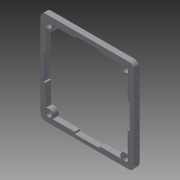
# Autodesk Inventor part: keyboard_space_cad
Saved by Autodesk Inventor 2014 (Build 180170000, 170)
## iProperties
Created: 2014-07-19
Part Number: keyboard_space_cad
Material: Generic
Document SubType Name: Modeling
Designer: james
Density: 1 g/cm^3
Appearance: Default
Author: james
Autodesk Inventor part; units mm, degrees
ref_plane "YZ Plane" through (0, 0, 0) normal (1, 0, 0) x (0, 1, 0)
ref_plane "XZ Plane" through (0, 0, 0) normal (0, 1, 0) x (-1, 0, 0)
ref_plane "XY Plane" through (0, 0, 0) normal (0, 0, 1) x (1, 0, 0)
sketch "Baseline" plane through (0, 0, 0) normal (0, 1, 0) x (-1, 0, 0)
  line L0 (61.0726, -11.6756) -> (16.1384, -11.6756)
  spline S0 degree 3 poles (16.1384, -11.6756) (13.8101, -11.6756) (11.9051, -13.5806) (11.9051, -15.909) knots 1 1 1 1 2 2 2 2
  line L1 (16.1384, -11.6756) -> (13.8101, -11.6756) construction
  line L2 (13.8101, -11.6756) -> (11.9051, -13.5806) construction
  line L3 (11.9051, -13.5806) -> (11.9051, -15.909) construction
  line L4 (11.9051, -15.909) -> (11.9051, -60.661)
  spline S1 degree 3 poles (11.9051, -60.661) (11.9051, -62.9893) (13.8101, -64.8943) (16.1384, -64.8943) knots 3 3 3 3 4 4 4 4
  line L5 (11.9051, -60.661) -> (11.9051, -62.9893) construction
  line L6 (11.9051, -62.9893) -> (13.8101, -64.8943) construction
  line L7 (13.8101, -64.8943) -> (16.1384, -64.8943) construction
  line L8 (16.1384, -64.8943) -> (61.0726, -64.8943)
  spline S2 degree 3 poles (61.0726, -64.8943) (63.4009, -64.8943) (65.3059, -62.9893) (65.3059, -60.661) knots 5 5 5 5 6 6 6 6
  line L9 (61.0726, -64.8943) -> (63.4009, -64.8943) construction
  line L10 (63.4009, -64.8943) -> (65.3059, -62.9893) construction
  line L11 (65.3059, -62.9893) -> (65.3059, -60.661) construction
  line L12 (65.3059, -60.661) -> (65.3059, -15.909)
  spline S3 degree 3 poles (65.3059, -15.909) (65.3059, -13.5806) (63.4009, -11.6756) (61.0726, -11.6756) knots 7 7 7 7 8 8 8 8
  line L13 (65.3059, -15.909) -> (65.3059, -13.5806) construction
  line L14 (65.3059, -13.5806) -> (63.4009, -11.6756) construction
  line L15 (63.4009, -11.6756) -> (61.0726, -11.6756) construction
  spline S4 degree 3 poles (59.9166, -15.3859) (59.9168, -15.3857) (59.9171, -15.3855) (59.9173, -15.3853) knots 0 0 0 0 1 1 1 1
  line L16 (59.9166, -15.3859) -> (59.9168, -15.3857) construction
  line L17 (59.9168, -15.3857) -> (59.9171, -15.3855) construction
  line L18 (59.9171, -15.3855) -> (59.9173, -15.3853) construction
  line L19 (59.9173, -15.3853) -> (59.9173, -15.3854)
  spline S5 degree 3 poles (59.9173, -15.3854) (60.1545, -15.1997) (60.4494, -15.0845) (60.7739, -15.0845) (61.5454, -15.0845) (62.1709, -15.7099) (62.1709, -16.4815) (62.1709, -16.7261) (62.1024, -16.9527) (61.9919, -17.1527) knots 2 2 2 2 3 3 3 4 4 4 5 5 5 5
  line L20 (59.9173, -15.3854) -> (60.1545, -15.1997) construction
  line L21 (60.1545, -15.1997) -> (60.4494, -15.0845) construction
  line L22 (60.4494, -15.0845) -> (60.7739, -15.0845) construction
  line L23 (60.7739, -15.0845) -> (61.5454, -15.0845) construction
  line L24 (61.5454, -15.0845) -> (62.1709, -15.7099) construction
  line L25 (62.1709, -15.7099) -> (62.1709, -16.4815) construction
  line L26 (62.1709, -16.4815) -> (62.1709, -16.7261) construction
  line L27 (62.1709, -16.7261) -> (62.1024, -16.9527) construction
  line L28 (62.1024, -16.9527) -> (61.9919, -17.1527) construction
  line L29 (61.9919, -17.1527) -> (61.9919, -17.1527)
  spline S6 degree 3 poles (61.9919, -17.1527) (61.9084, -17.3039) (61.7991, -17.4365) (61.6678, -17.5468) knots 7 7 7 7 8 8 8 8
  line L30 (61.9919, -17.1527) -> (61.9084, -17.3039) construction
  line L31 (61.9084, -17.3039) -> (61.7991, -17.4365) construction
  line L32 (61.7991, -17.4365) -> (61.6678, -17.5468) construction
  spline S7 degree 3 poles (61.6678, -17.5468) (61.6518, -17.5604) (61.6359, -17.5739) (61.6194, -17.5867) knots 8 8 8 8 9 9 9 9
  line L33 (61.6678, -17.5468) -> (61.6518, -17.5604) construction
  line L34 (61.6518, -17.5604) -> (61.6359, -17.5739) construction
  line L35 (61.6359, -17.5739) -> (61.6194, -17.5867) construction
  spline S8 degree 3 poles (61.6194, -17.5867) (61.583, -17.6147) (61.5464, -17.6415) (61.5073, -17.6658) knots 9 9 9 9 10 10 10 10
  line L36 (61.6194, -17.5867) -> (61.583, -17.6147) construction
  line L37 (61.583, -17.6147) -> (61.5464, -17.6415) construction
  line L38 (61.5464, -17.6415) -> (61.5073, -17.6658) construction
  spline S9 degree 3 poles (61.5073, -17.6658) (61.4604, -17.6954) (61.4112, -17.7214) (61.3608, -17.7453) knots 10 10 10 10 11 11 11 11
  line L39 (61.5073, -17.6658) -> (61.4604, -17.6954) construction
  line L40 (61.4604, -17.6954) -> (61.4112, -17.7214) construction
  line L41 (61.4112, -17.7214) -> (61.3608, -17.7453) construction
  spline S10 degree 3 poles (61.3608, -17.7453) (61.3302, -17.7595) (61.2994, -17.7722) (61.2677, -17.7842) knots 11 11 11 11 12 12 12 12
  line L42 (61.3608, -17.7453) -> (61.3302, -17.7595) construction
  line L43 (61.3302, -17.7595) -> (61.2994, -17.7722) construction
  line L44 (61.2994, -17.7722) -> (61.2677, -17.7842) construction
  spline S11 degree 3 poles (61.2677, -17.7842) (61.2113, -17.8059) (61.1534, -17.824) (61.0936, -17.8382) knots 12 12 12 12 13 13 13 13
  line L45 (61.2677, -17.7842) -> (61.2113, -17.8059) construction
  line L46 (61.2113, -17.8059) -> (61.1534, -17.824) construction
  line L47 (61.1534, -17.824) -> (61.0936, -17.8382) construction
  spline S12 degree 3 poles (61.0936, -17.8382) (61.0698, -17.8439) (61.0461, -17.8491) (61.0217, -17.8535) knots 13 13 13 13 14 14 14 14
  line L48 (61.0936, -17.8382) -> (61.0698, -17.8439) construction
  line L49 (61.0698, -17.8439) -> (61.0461, -17.8491) construction
  line L50 (61.0461, -17.8491) -> (61.0217, -17.8535) construction
  spline S13 degree 3 poles (61.0217, -17.8535) (60.9411, -17.8682) (60.8589, -17.8785) (60.7739, -17.8785) (60.0023, -17.8785) (59.3769, -17.253) (59.3769, -16.4815) (59.3769, -16.3956) (59.387, -16.3124) (59.4021, -16.2311) knots 14 14 14 14 15 15 15 16 16 16 17 17 17 17
  line L51 (61.0217, -17.8535) -> (60.9411, -17.8682) construction
  line L52 (60.9411, -17.8682) -> (60.8589, -17.8785) construction
  line L53 (60.8589, -17.8785) -> (60.7739, -17.8785) construction
  line L54 (60.7739, -17.8785) -> (60.0023, -17.8785) construction
  line L55 (60.0023, -17.8785) -> (59.3769, -17.253) construction
  line L56 (59.3769, -17.253) -> (59.3769, -16.4815) construction
  line L57 (59.3769, -16.4815) -> (59.3769, -16.3956) construction
  line L58 (59.3769, -16.3956) -> (59.387, -16.3124) construction
  line L59 (59.387, -16.3124) -> (59.4021, -16.2311) construction
  spline S14 degree 3 poles (59.4021, -16.2311) (59.4052, -16.2142) (59.4075, -16.1974) (59.4112, -16.1808) knots 17 17 17 17 18 18 18 18
  line L60 (59.4021, -16.2311) -> (59.4052, -16.2142) construction
  line L61 (59.4052, -16.2142) -> (59.4075, -16.1974) construction
  line L62 (59.4075, -16.1974) -> (59.4112, -16.1808) construction
  spline S15 degree 3 poles (59.4112, -16.1808) (59.4271, -16.11) (59.4487, -16.0414) (59.475, -15.9752) knots 18 18 18 18 19 19 19 19
  line L63 (59.4112, -16.1808) -> (59.4271, -16.11) construction
  line L64 (59.4271, -16.11) -> (59.4487, -16.0414) construction
  line L65 (59.4487, -16.0414) -> (59.475, -15.9752) construction
  spline S16 degree 3 poles (59.475, -15.9752) (59.486, -15.9472) (59.4982, -15.9203) (59.5108, -15.8933) knots 19 19 19 19 20 20 20 20
  line L66 (59.475, -15.9752) -> (59.486, -15.9472) construction
  line L67 (59.486, -15.9472) -> (59.4982, -15.9203) construction
  line L68 (59.4982, -15.9203) -> (59.5108, -15.8933) construction
  spline S17 degree 3 poles (59.5108, -15.8933) (59.5311, -15.8506) (59.5537, -15.8095) (59.5781, -15.7694) knots 20 20 20 20 21 21 21 21
  line L69 (59.5108, -15.8933) -> (59.5311, -15.8506) construction
  line L70 (59.5311, -15.8506) -> (59.5537, -15.8095) construction
  line L71 (59.5537, -15.8095) -> (59.5781, -15.7694) construction
  spline S18 degree 3 poles (59.5781, -15.7694) (59.6085, -15.7183) (59.6422, -15.6703) (59.6788, -15.6237) knots 21 21 21 21 22 22 22 22
  line L72 (59.5781, -15.7694) -> (59.6085, -15.7183) construction
  line L73 (59.6085, -15.7183) -> (59.6422, -15.6703) construction
  line L74 (59.6422, -15.6703) -> (59.6788, -15.6237) construction
  spline S19 degree 3 poles (59.6788, -15.6237) (59.69, -15.6095) (59.7015, -15.5956) (59.7133, -15.5819) knots 22 22 22 22 23 23 23 23
  line L75 (59.6788, -15.6237) -> (59.69, -15.6095) construction
  line L76 (59.69, -15.6095) -> (59.7015, -15.5956) construction
  line L77 (59.7015, -15.5956) -> (59.7133, -15.5819) construction
  spline S20 degree 3 poles (59.7133, -15.5819) (59.7745, -15.5098) (59.8421, -15.4444) (59.9166, -15.3859) knots 23 23 23 23 24 24 24 24
  line L78 (59.7133, -15.5819) -> (59.7745, -15.5098) construction
  line L79 (59.7745, -15.5098) -> (59.8421, -15.4444) construction
  line L80 (59.8421, -15.4444) -> (59.9166, -15.3859) construction
  spline S21 degree 3 poles (16.8742, -15.0845) (17.2556, -15.0845) (17.6005, -15.2381) (17.8525, -15.4858) knots 0 0 0 0 1 1 1 1
  line L81 (16.8742, -15.0845) -> (17.2556, -15.0845) construction
  line L82 (17.2556, -15.0845) -> (17.6005, -15.2381) construction
  line L83 (17.6005, -15.2381) -> (17.8525, -15.4858) construction
  line L84 (17.8525, -15.4858) -> (17.8526, -15.4858)
  spline S22 degree 3 poles (17.8526, -15.4858) (17.8526, -15.4858) (17.8526, -15.4859) (17.8526, -15.4859) knots 2 2 2 2 3 3 3 3
  line L85 (17.8526, -15.4858) -> (17.8526, -15.4858) construction
  line L86 (17.8526, -15.4858) -> (17.8526, -15.4859) construction
  line L87 (17.8526, -15.4859) -> (17.8526, -15.4859) construction
  spline S23 degree 3 poles (17.8526, -15.4859) (17.9793, -15.6103) (18.0817, -15.7586) (18.1538, -15.9236) knots 3 3 3 3 4 4 4 4
  line L88 (17.8526, -15.4859) -> (17.9793, -15.6103) construction
  line L89 (17.9793, -15.6103) -> (18.0817, -15.7586) construction
  line L90 (18.0817, -15.7586) -> (18.1538, -15.9236) construction
  spline S24 degree 3 poles (18.1538, -15.9236) (18.1552, -15.9268) (18.1574, -15.9295) (18.1587, -15.9327) knots 4 4 4 4 5 5 5 5
  line L91 (18.1538, -15.9236) -> (18.1552, -15.9268) construction
  line L92 (18.1552, -15.9268) -> (18.1574, -15.9295) construction
  line L93 (18.1574, -15.9295) -> (18.1587, -15.9327) construction
  spline S25 degree 3 poles (18.1587, -15.9327) (18.1905, -16.0071) (18.2137, -16.0857) (18.2323, -16.166) knots 5 5 5 5 6 6 6 6
  line L94 (18.1587, -15.9327) -> (18.1905, -16.0071) construction
  line L95 (18.1905, -16.0071) -> (18.2137, -16.0857) construction
  line L96 (18.2137, -16.0857) -> (18.2323, -16.166) construction
  spline S26 degree 3 poles (18.2323, -16.166) (18.2348, -16.1769) (18.2399, -16.1867) (18.2422, -16.1977) knots 6 6 6 6 7 7 7 7
  line L97 (18.2323, -16.166) -> (18.2348, -16.1769) construction
  line L98 (18.2348, -16.1769) -> (18.2399, -16.1867) construction
  line L99 (18.2399, -16.1867) -> (18.2422, -16.1977) construction
  spline S27 degree 3 poles (18.2422, -16.1977) (18.2611, -16.2893) (18.2712, -16.3842) (18.2712, -16.4815) (18.2712, -16.8672) (18.1149, -17.2165) (17.8621, -17.4693) knots 7 7 7 7 8 8 8 9 9 9 9
  line L100 (18.2422, -16.1977) -> (18.2611, -16.2893) construction
  line L101 (18.2611, -16.2893) -> (18.2712, -16.3842) construction
  line L102 (18.2712, -16.3842) -> (18.2712, -16.4815) construction
  line L103 (18.2712, -16.4815) -> (18.2712, -16.8672) construction
  line L104 (18.2712, -16.8672) -> (18.1149, -17.2165) construction
  line L105 (18.1149, -17.2165) -> (17.8621, -17.4693) construction
  spline S28 degree 3 poles (17.8621, -17.4693) (17.6725, -17.6589) (17.4286, -17.7943) (17.1558, -17.8501) knots 9 9 9 9 10 10 10 10
  line L106 (17.8621, -17.4693) -> (17.6725, -17.6589) construction
  line L107 (17.6725, -17.6589) -> (17.4286, -17.7943) construction
  line L108 (17.4286, -17.7943) -> (17.1558, -17.8501) construction
  spline S29 degree 3 poles (17.1558, -17.8501) (17.0648, -17.8687) (16.9707, -17.8785) (16.8742, -17.8785) (16.7745, -17.8785) (16.6776, -17.8672) (16.5839, -17.8474) knots 10 10 10 10 11 11 11 12 12 12 12
  line L109 (17.1558, -17.8501) -> (17.0648, -17.8687) construction
  line L110 (17.0648, -17.8687) -> (16.9707, -17.8785) construction
  line L111 (16.9707, -17.8785) -> (16.8742, -17.8785) construction
  line L112 (16.8742, -17.8785) -> (16.7745, -17.8785) construction
  line L113 (16.7745, -17.8785) -> (16.6776, -17.8672) construction
  line L114 (16.6776, -17.8672) -> (16.5839, -17.8474) construction
  spline S30 degree 3 poles (16.5839, -17.8474) (16.5698, -17.8443) (16.5571, -17.8382) (16.5433, -17.8348) knots 12 12 12 12 13 13 13 13
  line L115 (16.5839, -17.8474) -> (16.5698, -17.8443) construction
  line L116 (16.5698, -17.8443) -> (16.5571, -17.8382) construction
  line L117 (16.5571, -17.8382) -> (16.5433, -17.8348) construction
  spline S31 degree 3 poles (16.5433, -17.8348) (16.4629, -17.8152) (16.3847, -17.7907) (16.3105, -17.7579) knots 13 13 13 13 14 14 14 14
  line L118 (16.5433, -17.8348) -> (16.4629, -17.8152) construction
  line L119 (16.4629, -17.8152) -> (16.3847, -17.7907) construction
  line L120 (16.3847, -17.7907) -> (16.3105, -17.7579) construction
  spline S32 degree 3 poles (16.3105, -17.7579) (16.3052, -17.7555) (16.3005, -17.752) (16.2952, -17.7496) knots 14 14 14 14 15 15 15 15
  line L121 (16.3105, -17.7579) -> (16.3052, -17.7555) construction
  line L122 (16.3052, -17.7555) -> (16.3005, -17.752) construction
  line L123 (16.3005, -17.752) -> (16.2952, -17.7496) construction
  spline S33 degree 3 poles (16.2952, -17.7496) (16.1272, -17.6727) (15.9783, -17.5637) (15.8541, -17.4302) knots 15 15 15 15 16 16 16 16
  line L124 (16.2952, -17.7496) -> (16.1272, -17.6727) construction
  line L125 (16.1272, -17.6727) -> (15.9783, -17.5637) construction
  line L126 (15.9783, -17.5637) -> (15.8541, -17.4302) construction
  spline S34 degree 3 poles (15.8541, -17.4302) (15.6221, -17.1808) (15.4772, -16.849) (15.4772, -16.4815) (15.4772, -15.7099) (16.1027, -15.0845) (16.8742, -15.0845) knots 18 18 18 18 19 19 19 20 20 20 20
  line L127 (15.8541, -17.4302) -> (15.6221, -17.1808) construction
  line L128 (15.6221, -17.1808) -> (15.4772, -16.849) construction
  line L129 (15.4772, -16.849) -> (15.4772, -16.4815) construction
  line L130 (15.4772, -16.4815) -> (15.4772, -15.7099) construction
  line L131 (15.4772, -15.7099) -> (16.1027, -15.0845) construction
  line L132 (16.1027, -15.0845) -> (16.8742, -15.0845) construction
  line L133 (17.8793, -61.432) -> (17.8793, -61.4321)
  spline S35 degree 3 poles (17.8793, -61.4321) (17.6285, -61.6715) (17.2906, -61.8205) (16.9166, -61.8205) (16.145, -61.8205) (15.5195, -61.195) (15.5195, -60.4235) (15.5195, -59.9667) (15.742, -59.5649) (16.0811, -59.31) knots 2 2 2 2 3 3 3 4 4 4 5 5 5 5
  line L134 (17.8793, -61.4321) -> (17.6285, -61.6715) construction
  line L135 (17.6285, -61.6715) -> (17.2906, -61.8205) construction
  line L136 (17.2906, -61.8205) -> (16.9166, -61.8205) construction
  line L137 (16.9166, -61.8205) -> (16.145, -61.8205) construction
  line L138 (16.145, -61.8205) -> (15.5195, -61.195) construction
  line L139 (15.5195, -61.195) -> (15.5195, -60.4235) construction
  line L140 (15.5195, -60.4235) -> (15.5195, -59.9667) construction
  line L141 (15.5195, -59.9667) -> (15.742, -59.5649) construction
  line L142 (15.742, -59.5649) -> (16.0811, -59.31) construction
  spline S36 degree 3 poles (16.0811, -59.31) (16.0818, -59.3094) (16.0823, -59.3088) (16.0831, -59.3083) knots 5 5 5 5 6 6 6 6
  line L143 (16.0811, -59.31) -> (16.0818, -59.3094) construction
  line L144 (16.0818, -59.3094) -> (16.0823, -59.3088) construction
  line L145 (16.0823, -59.3088) -> (16.0831, -59.3083) construction
  spline S37 degree 3 poles (16.0831, -59.3083) (16.155, -59.2545) (16.2317, -59.2079) (16.3134, -59.1685) knots 6 6 6 6 7 7 7 7
  line L146 (16.0831, -59.3083) -> (16.155, -59.2545) construction
  line L147 (16.155, -59.2545) -> (16.2317, -59.2079) construction
  line L148 (16.2317, -59.2079) -> (16.3134, -59.1685) construction
  spline S38 degree 3 poles (16.3134, -59.1685) (16.3218, -59.1643) (16.3295, -59.1591) (16.3381, -59.1551) knots 7 7 7 7 8 8 8 8
  line L149 (16.3134, -59.1685) -> (16.3218, -59.1643) construction
  line L150 (16.3218, -59.1643) -> (16.3295, -59.1591) construction
  line L151 (16.3295, -59.1591) -> (16.3381, -59.1551) construction
  spline S39 degree 3 poles (16.3381, -59.1551) (16.412, -59.1213) (16.4898, -59.0956) (16.57, -59.075) knots 8 8 8 8 9 9 9 9
  line L152 (16.3381, -59.1551) -> (16.412, -59.1213) construction
  line L153 (16.412, -59.1213) -> (16.4898, -59.0956) construction
  line L154 (16.4898, -59.0956) -> (16.57, -59.075) construction
  spline S40 degree 3 poles (16.57, -59.075) (16.5869, -59.0706) (16.6024, -59.0635) (16.6196, -59.0597) knots 9 9 9 9 10 10 10 10
  line L155 (16.57, -59.075) -> (16.5869, -59.0706) construction
  line L156 (16.5869, -59.0706) -> (16.6024, -59.0635) construction
  line L157 (16.6024, -59.0635) -> (16.6196, -59.0597) construction
  spline S41 degree 3 poles (16.6196, -59.0597) (16.7155, -59.0389) (16.8144, -59.0265) (16.9166, -59.0265) (17.013, -59.0265) (17.1072, -59.0363) (17.1981, -59.0549) knots 10 10 10 10 11 11 11 12 12 12 12
  line L158 (16.6196, -59.0597) -> (16.7155, -59.0389) construction
  line L159 (16.7155, -59.0389) -> (16.8144, -59.0265) construction
  line L160 (16.8144, -59.0265) -> (16.9166, -59.0265) construction
  line L161 (16.9166, -59.0265) -> (17.013, -59.0265) construction
  line L162 (17.013, -59.0265) -> (17.1072, -59.0363) construction
  line L163 (17.1072, -59.0363) -> (17.1981, -59.0549) construction
  spline S42 degree 3 poles (17.1981, -59.0549) (17.4709, -59.1107) (17.7148, -59.246) (17.9044, -59.4357) (18.1572, -59.6885) (18.3136, -60.0377) (18.3136, -60.4235) (18.3136, -60.522) (18.3028, -60.618) (18.2834, -60.7107) knots 12 12 12 12 13 13 13 14 14 14 15 15 15 15
  line L164 (17.1981, -59.0549) -> (17.4709, -59.1107) construction
  line L165 (17.4709, -59.1107) -> (17.7148, -59.246) construction
  line L166 (17.7148, -59.246) -> (17.9044, -59.4357) construction
  line L167 (17.9044, -59.4357) -> (18.1572, -59.6885) construction
  line L168 (18.1572, -59.6885) -> (18.3136, -60.0377) construction
  line L169 (18.3136, -60.0377) -> (18.3136, -60.4235) construction
  line L170 (18.3136, -60.4235) -> (18.3136, -60.522) construction
  line L171 (18.3136, -60.522) -> (18.3028, -60.618) construction
  line L172 (18.3028, -60.618) -> (18.2834, -60.7107) construction
  spline S43 degree 3 poles (18.2834, -60.7107) (18.2806, -60.724) (18.2747, -60.736) (18.2715, -60.7491) knots 15 15 15 15 16 16 16 16
  line L173 (18.2834, -60.7107) -> (18.2806, -60.724) construction
  line L174 (18.2806, -60.724) -> (18.2747, -60.736) construction
  line L175 (18.2747, -60.736) -> (18.2715, -60.7491) construction
  spline S44 degree 3 poles (18.2715, -60.7491) (18.2524, -60.8288) (18.2288, -60.9066) (18.1967, -60.9803) knots 16 16 16 16 17 17 17 17
  line L176 (18.2715, -60.7491) -> (18.2524, -60.8288) construction
  line L177 (18.2524, -60.8288) -> (18.2288, -60.9066) construction
  line L178 (18.2288, -60.9066) -> (18.1967, -60.9803) construction
  spline S45 degree 3 poles (18.1967, -60.9803) (18.1948, -60.9846) (18.192, -60.9883) (18.19, -60.9926) knots 17 17 17 17 18 18 18 18
  line L179 (18.1967, -60.9803) -> (18.1948, -60.9846) construction
  line L180 (18.1948, -60.9846) -> (18.192, -60.9883) construction
  line L181 (18.192, -60.9883) -> (18.19, -60.9926) construction
  spline S46 degree 3 poles (18.19, -60.9926) (18.1154, -61.1592) (18.0095, -61.3077) (17.8793, -61.432) knots 18 18 18 18 19 19 19 19
  line L182 (18.19, -60.9926) -> (18.1154, -61.1592) construction
  line L183 (18.1154, -61.1592) -> (18.0095, -61.3077) construction
  line L184 (18.0095, -61.3077) -> (17.8793, -61.432) construction
  spline S47 degree 3 poles (60.7739, -61.8205) (60.4493, -61.8205) (60.1545, -61.7053) (59.9173, -61.5196) knots 0 0 0 0 1 1 1 1
  line L185 (60.7739, -61.8205) -> (60.4493, -61.8205) construction
  line L186 (60.4493, -61.8205) -> (60.1545, -61.7053) construction
  line L187 (60.1545, -61.7053) -> (59.9173, -61.5196) construction
  line L188 (59.9173, -61.5196) -> (59.9171, -61.5194)
  spline S48 degree 3 poles (59.9171, -61.5194) (59.8423, -61.4608) (59.7745, -61.3953) (59.7131, -61.3229) knots 3 3 3 3 4 4 4 4
  line L189 (59.9171, -61.5194) -> (59.8423, -61.4608) construction
  line L190 (59.8423, -61.4608) -> (59.7745, -61.3953) construction
  line L191 (59.7745, -61.3953) -> (59.7131, -61.3229) construction
  spline S49 degree 3 poles (59.7131, -61.3229) (59.7014, -61.3093) (59.6901, -61.2955) (59.6789, -61.2815) knots 4 4 4 4 5 5 5 5
  line L192 (59.7131, -61.3229) -> (59.7014, -61.3093) construction
  line L193 (59.7014, -61.3093) -> (59.6901, -61.2955) construction
  line L194 (59.6901, -61.2955) -> (59.6789, -61.2815) construction
  spline S50 degree 3 poles (59.6789, -61.2815) (59.6422, -61.2347) (59.6084, -61.1865) (59.5778, -61.1352) knots 5 5 5 5 6 6 6 6
  line L195 (59.6789, -61.2815) -> (59.6422, -61.2347) construction
  line L196 (59.6422, -61.2347) -> (59.6084, -61.1865) construction
  line L197 (59.6084, -61.1865) -> (59.5778, -61.1352) construction
  spline S51 degree 3 poles (59.5778, -61.1352) (59.5536, -61.0952) (59.5311, -61.0543) (59.5109, -61.0119) knots 6 6 6 6 7 7 7 7
  line L198 (59.5778, -61.1352) -> (59.5536, -61.0952) construction
  line L199 (59.5536, -61.0952) -> (59.5311, -61.0543) construction
  line L200 (59.5311, -61.0543) -> (59.5109, -61.0119) construction
  spline S52 degree 3 poles (59.5109, -61.0119) (59.4982, -60.9847) (59.486, -60.9578) (59.475, -60.9298) knots 7 7 7 7 8 8 8 8
  line L201 (59.5109, -61.0119) -> (59.4982, -60.9847) construction
  line L202 (59.4982, -60.9847) -> (59.486, -60.9578) construction
  line L203 (59.486, -60.9578) -> (59.475, -60.9298) construction
  spline S53 degree 3 poles (59.475, -60.9298) (59.4487, -60.8635) (59.4271, -60.795) (59.4112, -60.7241) knots 8 8 8 8 9 9 9 9
  line L204 (59.475, -60.9298) -> (59.4487, -60.8635) construction
  line L205 (59.4487, -60.8635) -> (59.4271, -60.795) construction
  line L206 (59.4271, -60.795) -> (59.4112, -60.7241) construction
  spline S54 degree 3 poles (59.4112, -60.7241) (59.4075, -60.7075) (59.4052, -60.6907) (59.4021, -60.6739) knots 9 9 9 9 10 10 10 10
  line L207 (59.4112, -60.7241) -> (59.4075, -60.7075) construction
  line L208 (59.4075, -60.7075) -> (59.4052, -60.6907) construction
  line L209 (59.4052, -60.6907) -> (59.4021, -60.6739) construction
  spline S55 degree 3 poles (59.4021, -60.6739) (59.387, -60.5925) (59.3769, -60.5094) (59.3769, -60.4235) (59.3769, -59.6519) (60.0023, -59.0265) (60.7739, -59.0265) (60.8589, -59.0265) (60.9411, -59.0368) (61.0217, -59.0515) knots 10 10 10 10 11 11 11 12 12 12 13 13 13 13
  line L210 (59.4021, -60.6739) -> (59.387, -60.5925) construction
  line L211 (59.387, -60.5925) -> (59.3769, -60.5094) construction
  line L212 (59.3769, -60.5094) -> (59.3769, -60.4235) construction
  line L213 (59.3769, -60.4235) -> (59.3769, -59.6519) construction
  line L214 (59.3769, -59.6519) -> (60.0023, -59.0265) construction
  line L215 (60.0023, -59.0265) -> (60.7739, -59.0265) construction
  line L216 (60.7739, -59.0265) -> (60.8589, -59.0265) construction
  line L217 (60.8589, -59.0265) -> (60.9411, -59.0368) construction
  line L218 (60.9411, -59.0368) -> (61.0217, -59.0515) construction
  spline S56 degree 3 poles (61.0217, -59.0515) (61.0461, -59.0558) (61.0698, -59.0611) (61.0936, -59.0667) knots 13 13 13 13 14 14 14 14
  line L219 (61.0217, -59.0515) -> (61.0461, -59.0558) construction
  line L220 (61.0461, -59.0558) -> (61.0698, -59.0611) construction
  line L221 (61.0698, -59.0611) -> (61.0936, -59.0667) construction
  spline S57 degree 3 poles (61.0936, -59.0667) (61.1534, -59.081) (61.2113, -59.099) (61.2677, -59.1208) knots 14 14 14 14 15 15 15 15
  line L222 (61.0936, -59.0667) -> (61.1534, -59.081) construction
  line L223 (61.1534, -59.081) -> (61.2113, -59.099) construction
  line L224 (61.2113, -59.099) -> (61.2677, -59.1208) construction
  spline S58 degree 3 poles (61.2677, -59.1208) (61.2994, -59.1328) (61.3302, -59.1455) (61.3608, -59.1597) knots 15 15 15 15 16 16 16 16
  line L225 (61.2677, -59.1208) -> (61.2994, -59.1328) construction
  line L226 (61.2994, -59.1328) -> (61.3302, -59.1455) construction
  line L227 (61.3302, -59.1455) -> (61.3608, -59.1597) construction
  spline S59 degree 3 poles (61.3608, -59.1597) (61.4112, -59.1836) (61.4604, -59.2096) (61.5073, -59.2392) knots 16 16 16 16 17 17 17 17
  line L228 (61.3608, -59.1597) -> (61.4112, -59.1836) construction
  line L229 (61.4112, -59.1836) -> (61.4604, -59.2096) construction
  line L230 (61.4604, -59.2096) -> (61.5073, -59.2392) construction
  spline S60 degree 3 poles (61.5073, -59.2392) (61.5464, -59.2635) (61.583, -59.2903) (61.6194, -59.3182) knots 17 17 17 17 18 18 18 18
  line L231 (61.5073, -59.2392) -> (61.5464, -59.2635) construction
  line L232 (61.5464, -59.2635) -> (61.583, -59.2903) construction
  line L233 (61.583, -59.2903) -> (61.6194, -59.3182) construction
  spline S61 degree 3 poles (61.6194, -59.3182) (61.6359, -59.3311) (61.6518, -59.3446) (61.6678, -59.3581) knots 18 18 18 18 19 19 19 19
  line L234 (61.6194, -59.3182) -> (61.6359, -59.3311) construction
  line L235 (61.6359, -59.3311) -> (61.6518, -59.3446) construction
  line L236 (61.6518, -59.3446) -> (61.6678, -59.3581) construction
  spline S62 degree 3 poles (61.6678, -59.3581) (61.7991, -59.4685) (61.9084, -59.6011) (61.9919, -59.7522) knots 19 19 19 19 20 20 20 20
  line L237 (61.6678, -59.3581) -> (61.7991, -59.4685) construction
  line L238 (61.7991, -59.4685) -> (61.9084, -59.6011) construction
  line L239 (61.9084, -59.6011) -> (61.9919, -59.7522) construction
  spline S63 degree 3 poles (61.9919, -59.7522) (61.9919, -59.7522) (61.9919, -59.7523) (61.9919, -59.7523) knots 20 20 20 20 21 21 21 21
  line L240 (61.9919, -59.7522) -> (61.9919, -59.7522) construction
  line L241 (61.9919, -59.7522) -> (61.9919, -59.7523) construction
  line L242 (61.9919, -59.7523) -> (61.9919, -59.7523) construction
  spline S64 degree 3 poles (61.9919, -59.7523) (62.1024, -59.9523) (62.1709, -60.1788) (62.1709, -60.4235) (62.1709, -61.195) (61.5454, -61.8205) (60.7739, -61.8205) knots 22 22 22 22 23 23 23 24 24 24 24
  line L243 (61.9919, -59.7523) -> (62.1024, -59.9523) construction
  line L244 (62.1024, -59.9523) -> (62.1709, -60.1788) construction
  line L245 (62.1709, -60.1788) -> (62.1709, -60.4235) construction
  line L246 (62.1709, -60.4235) -> (62.1709, -61.195) construction
  line L247 (62.1709, -61.195) -> (61.5454, -61.8205) construction
  line L248 (61.5454, -61.8205) -> (60.7739, -61.8205) construction
  spline S65 degree 3 poles (62.5971, -57.5872) (62.5971, -57.8109) (62.5744, -58.029) (62.5405, -58.2435) knots 0 0 0 0 1 1 1 1
  line L249 (62.5971, -57.5872) -> (62.5971, -57.8109) construction
  line L250 (62.5971, -57.8109) -> (62.5744, -58.029) construction
  line L251 (62.5744, -58.029) -> (62.5405, -58.2435) construction
  spline S66 degree 3 poles (62.5405, -58.2435) (62.0576, -57.8514) (61.443, -57.6154) (60.7739, -57.6154) (59.2255, -57.6154) (57.9658, -58.8751) (57.9658, -60.4235) (57.9658, -60.9323) (58.1039, -61.4085) (58.3414, -61.8205) knots 1 1 1 1 2 2 2 3 3 3 4 4 4 4
  line L252 (62.5405, -58.2435) -> (62.0576, -57.8514) construction
  line L253 (62.0576, -57.8514) -> (61.443, -57.6154) construction
  line L254 (61.443, -57.6154) -> (60.7739, -57.6154) construction
  line L255 (60.7739, -57.6154) -> (59.2255, -57.6154) construction
  line L256 (59.2255, -57.6154) -> (57.9658, -58.8751) construction
  line L257 (57.9658, -58.8751) -> (57.9658, -60.4235) construction
  line L258 (57.9658, -60.4235) -> (57.9658, -60.9323) construction
  line L259 (57.9658, -60.9323) -> (58.1039, -61.4085) construction
  line L260 (58.1039, -61.4085) -> (58.3414, -61.8205) construction
  line L261 (58.3414, -61.8205) -> (19.6354, -61.8205)
  spline S67 degree 3 poles (19.6354, -61.8205) (19.5417, -61.8205) (19.4499, -61.8124) (19.3576, -61.8064) knots 5 5 5 5 6 6 6 6
  line L262 (19.6354, -61.8205) -> (19.5417, -61.8205) construction
  line L263 (19.5417, -61.8205) -> (19.4499, -61.8124) construction
  line L264 (19.4499, -61.8124) -> (19.3576, -61.8064) construction
  spline S68 degree 3 poles (19.3576, -61.8064) (19.5901, -61.3976) (19.7247, -60.9264) (19.7247, -60.4235) (19.7247, -58.8751) (18.465, -57.6154) (16.9166, -57.6154) (16.3697, -57.6154) (15.8605, -57.775) (15.4284, -58.0465) knots 6 6 6 6 7 7 7 8 8 8 9 9 9 9
  line L265 (19.3576, -61.8064) -> (19.5901, -61.3976) construction
  line L266 (19.5901, -61.3976) -> (19.7247, -60.9264) construction
  line L267 (19.7247, -60.9264) -> (19.7247, -60.4235) construction
  line L268 (19.7247, -60.4235) -> (19.7247, -58.8751) construction
  line L269 (19.7247, -58.8751) -> (18.465, -57.6154) construction
  line L270 (18.465, -57.6154) -> (16.9166, -57.6154) construction
  line L271 (16.9166, -57.6154) -> (16.3697, -57.6154) construction
  line L272 (16.3697, -57.6154) -> (15.8605, -57.775) construction
  line L273 (15.8605, -57.775) -> (15.4284, -58.0465) construction
  spline S69 degree 3 poles (15.4284, -58.0465) (15.4119, -57.8954) (15.4021, -57.7424) (15.4021, -57.5872) knots 9 9 9 9 10 10 10 10
  line L274 (15.4284, -58.0465) -> (15.4119, -57.8954) construction
  line L275 (15.4119, -57.8954) -> (15.4021, -57.7424) construction
  line L276 (15.4021, -57.7424) -> (15.4021, -57.5872) construction
  line L277 (15.4021, -57.5872) -> (15.4021, -19.3178)
  spline S70 degree 3 poles (15.4021, -19.3178) (15.4021, -19.1707) (15.4099, -19.0254) (15.4248, -18.882) knots 11 11 11 11 12 12 12 12
  line L278 (15.4021, -19.3178) -> (15.4021, -19.1707) construction
  line L279 (15.4021, -19.1707) -> (15.4099, -19.0254) construction
  line L280 (15.4099, -19.0254) -> (15.4248, -18.882) construction
  spline S71 degree 3 poles (15.4248, -18.882) (15.8486, -19.1389) (16.3435, -19.2896) (16.8742, -19.2896) (18.4226, -19.2896) (19.6823, -18.0299) (19.6823, -16.4815) (19.6823, -15.9795) (19.5483, -15.5089) (19.3165, -15.1007) knots 12 12 12 12 13 13 13 14 14 14 15 15 15 15
  line L281 (15.4248, -18.882) -> (15.8486, -19.1389) construction
  line L282 (15.8486, -19.1389) -> (16.3435, -19.2896) construction
  line L283 (16.3435, -19.2896) -> (16.8742, -19.2896) construction
  line L284 (16.8742, -19.2896) -> (18.4226, -19.2896) construction
  line L285 (18.4226, -19.2896) -> (19.6823, -18.0299) construction
  line L286 (19.6823, -18.0299) -> (19.6823, -16.4815) construction
  line L287 (19.6823, -16.4815) -> (19.6823, -15.9795) construction
  line L288 (19.6823, -15.9795) -> (19.5483, -15.5089) construction
  line L289 (19.5483, -15.5089) -> (19.3165, -15.1007) construction
  spline S72 degree 3 poles (19.3165, -15.1007) (19.4222, -15.0927) (19.5278, -15.0845) (19.6354, -15.0845) knots 15 15 15 15 16 16 16 16
  line L290 (19.3165, -15.1007) -> (19.4222, -15.0927) construction
  line L291 (19.4222, -15.0927) -> (19.5278, -15.0845) construction
  line L292 (19.5278, -15.0845) -> (19.6354, -15.0845) construction
  spline S73 degree 3 poles (58.3414, -15.0845) (58.1039, -15.4965) (57.9658, -15.9727) (57.9658, -16.4815) (57.9658, -18.0299) (59.2255, -19.2896) (60.7739, -19.2896) (61.443, -19.2896) (62.0576, -19.0536) (62.5405, -18.6614) knots 17 17 17 17 18 18 18 19 19 19 20 20 20 20
  line L293 (58.3414, -15.0845) -> (58.1039, -15.4965) construction
  line L294 (58.1039, -15.4965) -> (57.9658, -15.9727) construction
  line L295 (57.9658, -15.9727) -> (57.9658, -16.4815) construction
  line L296 (57.9658, -16.4815) -> (57.9658, -18.0299) construction
  line L297 (57.9658, -18.0299) -> (59.2255, -19.2896) construction
  line L298 (59.2255, -19.2896) -> (60.7739, -19.2896) construction
  line L299 (60.7739, -19.2896) -> (61.443, -19.2896) construction
  line L300 (61.443, -19.2896) -> (62.0576, -19.0536) construction
  line L301 (62.0576, -19.0536) -> (62.5405, -18.6614) construction
  spline S74 degree 3 poles (62.5405, -18.6614) (62.5744, -18.876) (62.5971, -19.0941) (62.5971, -19.3178) knots 20 20 20 20 21 21 21 21
  line L302 (62.5405, -18.6614) -> (62.5744, -18.876) construction
  line L303 (62.5744, -18.876) -> (62.5971, -19.0941) construction
  line L304 (62.5971, -19.0941) -> (62.5971, -19.3178) construction
  line L305 (62.5989, -19.3178) -> (62.6148, -57.5872)
  point P0 (0, 0)
  constraints: 24 end point, 225 other
sketch "Sketch2" plane through (0, 0, 0) normal (0, 1, 0) x (-1, 0, 0)
  arc A0 (15.4198, -18.8831) -> (19.312, -15.1063) centre (16.8686, -16.4822) ccw
  arc A1 (19.312, -61.8046) -> (15.4198, -58.0465) centre (16.9261, -60.381) ccw
  arc A2 (62.5444, -58.244) -> (58.3471, -61.8046) centre (60.767, -60.4029) ccw
  arc A3 (58.3471, -15.1063) -> (62.5444, -18.6734) centre (60.7755, -16.5019) ccw
  line L0 (62.4312, -11.5226) -> (14.8247, -11.5226)
  line L1 (11.8247, -14.5226) -> (11.8247, -61.8396)
  line L2 (14.8247, -64.8396) -> (62.4312, -64.8396)
  line L3 (65.4312, -61.8396) -> (65.4312, -14.5226)
  arc A4 (62.4312, -64.8396) -> (65.4312, -61.8396) centre (62.4312, -61.8396) ccw
  arc A5 (11.8247, -61.8396) -> (14.8247, -64.8396) centre (14.8247, -61.8396) ccw
  arc A6 (14.8247, -11.5226) -> (11.8247, -14.5226) centre (14.8247, -14.5226) ccw
  arc A7 (65.4312, -14.5226) -> (62.4312, -11.5226) centre (62.4312, -14.5226) ccw
  line L4 (58.3471, -15.1063) -> (45.232, -15.1063)
  line L5 (19.312, -15.1063) -> (31.812, -15.1063)
  line L6 (31.812, -15.1063) -> (31.812, -14.1063)
  line L7 (31.812, -14.1063) -> (45.232, -14.1063)
  line L8 (45.232, -14.1063) -> (45.232, -15.1063)
  line L9 (15.4198, -18.8831) -> (15.4198, -31.3831)
  line L10 (15.4198, -31.3831) -> (14.4198, -31.3831)
  line L11 (15.4198, -58.0465) -> (15.4198, -45.5465)
  line L12 (15.4198, -45.5465) -> (14.4198, -45.5465)
  line L13 (14.4198, -45.5465) -> (14.4198, -31.3831)
  line L14 (19.312, -61.8046) -> (31.812, -61.8046)
  line L15 (58.3471, -61.8046) -> (45.8471, -61.8046)
  line L16 (45.8471, -61.8046) -> (45.8471, -62.8046)
  line L17 (45.8471, -62.8046) -> (31.812, -62.8046)
  line L18 (31.812, -62.8046) -> (31.812, -61.8046)
  line L19 (62.5444, -18.6734) -> (62.5444, -31.1734)
  line L20 (62.5444, -58.244) -> (62.5444, -45.744)
  line L21 (62.5444, -45.744) -> (63.5444, -45.744)
  line L22 (63.5444, -45.744) -> (63.5444, -31.1734)
  line L23 (63.5444, -31.1734) -> (62.5444, -31.1734)
  circle A8 centre (60.7791, -16.4067) radius 1.55
  circle A9 centre (60.767, -60.4029) radius 1.55
  circle A10 centre (16.7694, -60.4038) radius 1.55
  circle A11 centre (16.7694, -16.4067) radius 1.55
  point P0 (0, 0)
  dimension "d1" = 3
  dimension "d2" = 3
  dimension "d8" = 47.6065
  dimension "d11" = 12.5
  dimension "d12" = 1
  dimension "d13" = 12.5
  dimension "d14" = 1
  dimension "d15" = 12.5
  dimension "d16" = 12.5
  dimension "d17" = 12.5
  dimension "d18" = 1
  dimension "d19" = 12.5
  dimension "d20" = 12.5
  dimension "d21" = 1
  dimension "d22" = 3.1
  dimension "d24" = 53.6065
  dimension "d25" = 3.1
  dimension "d26" = 3.1
  dimension "d27" = 3.1
  constraints: 48 end point, 16 point on circle, 12 centre point, 10 parallel, 9 perpendicular, 8 tangent, 3 collinear, 2 equal radius, 1 coincident, 1 horizontal
  measures "d1" radius of A4
  measures "d2" radius of A7
  measures "d8" distance of L0.start L0.end
  measures "d11" distance of L5.start L5.end
  measures "d12" distance of L5.end L6.end
  measures "d13" distance of L9.start L9.end
  measures "d14" distance of L9.end L10.end
  measures "d15" distance of L11.start L11.end
  measures "d16" distance of L14.start L14.end
  measures "d17" distance of L15.start L15.end
  measures "d18" distance of L15.end L16.end
  measures "d19" distance of L19.start L19.end
  measures "d20" distance of L20.start L20.end
  measures "d21" distance of L20.end L21.end
  measures "d22" diameter of A8
  measures "d24" distance between parallel lines of L3 L1
  measures "d25" diameter of A9
  measures "d26" diameter of A10
  measures "d27" diameter of A11
extrude "Extrusion2" add sketch "Sketch2" along normal blind 3.1
body "Solid2"
